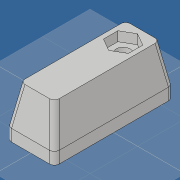
# Autodesk Inventor part: Verschluss_Knauf
Saved by Autodesk Inventor 2019 (Build 230136000, 136)
## iProperties
Created: 2020-08-31
Part Number: Verschluss_Knauf
Material: Generisch
Document SubType Name: Modeling
Designer: Stefan
Mass: 15.7698 g
Surface Area: 50.4939 cm^2
Volume: 15.7698 cm^3
Density: 1 g/cm^3
Appearance: Vorgabe
Author: Stefan
Autodesk Inventor part; units mm, degrees
ref_plane "YZ Plane" through (0, 0, 0) normal (1, 0, 0) x (0, 1, 0)
ref_plane "XZ Plane" through (0, 0, 0) normal (0, 1, 0) x (-1, 0, 0)
ref_plane "XY Plane" through (0, 0, 0) normal (0, 0, 1) x (1, 0, 0)
sketch "Skizze1" plane through (0, 0, 0) normal (0, 1, 0) x (-1, 0, 0)
  line L0 (-10, 25) -> (10, 25)
  line L1 (10, 25) -> (10, -25)
  line L2 (10, -25) -> (-10, -25)
  line L3 (-10, -25) -> (-10, 25)
  line L4 (-10, 25) -> (10, -25) construction
  line L5 (10, 25) -> (-10, -25) construction
  line L6 (0, -20) -> (-5.25, -16.9689)
  line L7 (-5.25, -16.9689) -> (-5.25, -10.9067)
  line L8 (-5.25, -10.9067) -> (0, -7.8756)
  line L9 (0, -7.8756) -> (5.25, -10.9067)
  line L10 (5.25, -10.9067) -> (5.25, -16.9689)
  line L11 (5.25, -16.9689) -> (0, -20)
  circle A0 centre (0, -13.9378) radius 3
  circle A1 centre (0, -13.9378) radius 6.0622
  point P0 (0, 0)
  point P1 (0, 0)
  dimension "d0" = 10.5
  dimension "d1" = 20
  dimension "d2" = 50
  dimension "d3" = 5
  dimension "d6" = 6
  constraints: 24 end point, 3 midpoint, 2 coincident, 2 parallel, 1 centre point, 1 horizontal, 1 perpendicular, 1 vertical, 1 vertical alignment, 16 other
  measures "d0" distance between parallel lines of L7 L10
  measures "d1" distance between parallel lines of L3 L1
  measures "d2" distance of L0.end L1.end
  measures "d3" distance from line of L2 L6.start
  measures "d6" diameter of A0
extrude "Extrusion1" add sketch "Skizze1" against normal blind 2 contours L0 L1 L2 L3 | A1 L6 | L6 L7 L8 L9 L10 L11 | L11 A1 | A1 L7 | L10 A1 | A1 L8 | L9 A1
extrude "Extrusion2" add sketch "Skizze1" along normal blind 4 contours L0 L1 L2 L3 | A1 L6 | L11 A1 | A1 L7 | L10 A1 | A1 L8 | L9 A1
extrude "Extrusion3" add sketch "Skizze1" against normal blind 17 contours L0 L1 L2 L3
sketch "Skizze2" plane through (0, 0, 0) normal (1, 0, 0) x (0, 1, 0)
  line L0 (0, -10.9378) -> (-2, -10.9378) projected
  line L1 (-2, -10.9378) -> (-2, -7.8756) projected
  line L2 (-2, -7.8756) -> (-17, -7.8756) projected
  line L3 (-17, -7.8756) -> (-17, 25) projected
  line L4 (-17, 25) -> (4, 25) projected
  line L5 (4, 25) -> (4, -7.8756) projected
  line L6 (4, -7.8756) -> (0, -7.8756) projected
  line L7 (0, -7.8756) -> (0, -10.9378) projected
  line L8 (-2, -16.9378) -> (0, -16.9378) projected
  line L9 (0, -16.9378) -> (0, -20) projected
  line L10 (0, -20) -> (4, -20) projected
  line L11 (4, -20) -> (4, -25) projected
  line L12 (4, -25) -> (-17, -25) projected
  line L13 (-17, -25) -> (-17, -20) projected
  line L14 (-17, -20) -> (-2, -20) projected
  line L15 (-2, -20) -> (-2, -16.9378) projected
  line L16 (-12, 25) -> (4, 22.1788)
  line L17 (4, 25) -> (4, 22.1788)
  line L18 (4, 25) -> (-12, 25)
  line L19 (4, -22.1788) -> (4, -25)
  line L20 (4, -22.1788) -> (-12, -25)
  line L21 (4, -25) -> (-12, -25)
  point P0 (0, 0)
  dimension "d12" = 5
  dimension "d13" = 10
  dimension "d14" = 10
  constraints: 12 end point, 4 point on line, 3 collinear, 1 perpendicular, 1 vertical alignment
  measures "d12" distance from line of L3 L16.start
  measures "d13" angle of L18 L16
  measures "d14" angle of L12 L20
extrude "Extrusion4" cut sketch "Skizze2" along normal through all both and the other way through all contours L16 L4 L5 | L11 L12 L20
sketch "Skizze3" plane through (0, 0, 0) normal (0, 0, 1) x (1, 0, 0)
  line L0 (-10, 4) -> (10, 4) projected
  line L1 (10, 4) -> (10, -17) projected
  line L2 (10, -17) -> (-10, -17) projected
  line L3 (-10, -17) -> (-10, 4) projected
  line L4 (-7.1788, 4) -> (-10, 4)
  line L5 (-10, -12) -> (-10, 4)
  line L6 (-10, -12) -> (-7.1788, 4)
  line L7 (7.1788, 4) -> (10, 4)
  line L8 (10, 4) -> (10, -12)
  line L9 (10, -12) -> (7.1788, 4)
  point P0 (0, 0)
  dimension "d17" = 10
  dimension "d18" = 10
  dimension "d19" = 5
  constraints: 12 end point, 4 point on line, 2 collinear, 1 horizontal alignment, 1 perpendicular
  measures "d17" angle of L3 L6
  measures "d18" angle of L1 L9
  measures "d19" distance from line of L2 L5.start
extrude "Extrusion5" cut sketch "Skizze3" along normal through all both and the other way through all contours L0 L6 L3 | L0 L1 L9
fillet "Rundung1" radius 2 8 edges at (8.5894, -4, 23.5894) (10, -14.5, 25) (-8.5894, -4, 23.5894) (-10, -14.5, 25) (-8.5894, -4, -23.5894) (-10, -14.5, -25) (8.5894, -4, -23.5894) (10, -14.5, -25)
equation "\"d18\" = d17"
equation "\"d19\" = d12"
